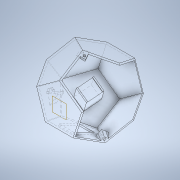
# Autodesk Inventor part: dodecahedron
Saved by Autodesk Inventor 2020.2 (Build 242310000, 310)
## iProperties
Created: 2020-01-17
Part Number: dodecahedron
Material: Generic
Document SubType Name: Modeling
Designer: Bardo91
Density: 1 g/cm^3
Appearance: Default
Author: Bardo91
Autodesk Inventor part; units mm, degrees
ref_plane "YZ Plane" through (0, 0, 0) normal (1, 0, 0) x (0, 1, 0)
ref_plane "XZ Plane" through (0, 0, 0) normal (0, 1, 0) x (-1, 0, 0)
ref_plane "Work Plane1" through (0, 0, 44.5407) normal (0, 0, 1) x (1, 0, 0)
sketch "Sketch2" plane through (0, 0, 44.5407) normal (0, 0, 1) x (1, 0, 0)
  line L0 (0, 34.026) -> (32.3607, 10.5146)
  line L1 (32.3607, 10.5146) -> (20, -27.5276)
  line L2 (20, -27.5276) -> (-20, -27.5276)
  line L3 (-20, -27.5276) -> (-32.3607, 10.5146)
  line L4 (-32.3607, 10.5146) -> (0, 34.026)
  point P0 (0, 0)
  point P1 (0, 0)
  dimension "d2" = 40
  constraints: 10 end point, 1 coincident, 11 other
  measures "d2" distance of L1.end L2.end
loft "Loft1" add profiles "Sketch2" section 2 point at (0, 0, 0)
mirror "Mirror1" about plane through (32.3607, 10.5146, 44.5407) normal (0.809017, -0.2628656, -0.5257311) of "Loft1"
mirror "Mirror2" about plane through (20, -27.5276, 44.5407) normal (0, -0.8506508, -0.5257311) of "Loft1"
mirror "Mirror3" about plane through (-20, -27.5276, 44.5407) normal (-0.809017, -0.2628656, -0.5257311) of "Loft1"
mirror "Mirror4" about plane through (-32.3607, 10.5146, 44.5407) normal (-0.5, 0.688191, -0.5257311) of "Loft1"
mirror "Mirror5" about plane through (0, 34.026, 44.5407) normal (0.5, 0.688191, -0.5257311) of "Loft1"
mirror "Mirror6" about plane through (-52.3607, -17.013, -10.5146) normal (0.309017, -0.4253254, -0.8506508) of "Loft1", "Mirror3"
mirror "Mirror7" about plane through (-52.3607, 17.013, 10.5146) normal (0, 0.5257311, -0.8506508) of "Loft1", "Mirror3"
mirror "Mirror8" about plane through (52.3607, -17.013, -10.5146) normal (0, 0.5257311, -0.8506508) of "Loft1", "Mirror1"
mirror "Mirror9" about plane through (20, 27.5276, -44.5407) normal (-0.809017, -0.2628656, -0.5257311) of "Loft1", "Mirror1", "Mirror8"
shell "Shell1" thickness 2 removed faces 3 at (21.5738, 29.6938, 26.1889) at (39.0273, 17.013, -14.8469) at (39.0273, -5.671, 21.8566)
sketch "Sketch3" plane through (-30.9076, -10.0425, -42.5407) normal (0.5257311, 0.7236068, 0.4472136) x (0.809017, -0.5877853, 0)
  line L0 (19.1019, -26.2916) -> (10.1019, -26.2916)
  line L1 (10.1019, -26.2916) -> (10.1019, -15.2916)
  line L2 (10.1019, -15.2916) -> (28.1019, -15.2916)
  line L3 (28.1019, -15.2916) -> (28.1019, -37.2916)
  line L4 (28.1019, -37.2916) -> (10.1019, -37.2916)
  line L5 (10.1019, -37.2916) -> (10.1019, -26.2916)
  dimension "d8" = 9
  dimension "d9" = 11
  dimension "d10" = 18
  dimension "d11" = 22
  constraints: 12 end point, 4 perpendicular, 1 horizontal, 1 point on line, 1 vertical
  measures "d8" distance of L0.start L0.end
  measures "d9" distance of L0.end L1.end
  measures "d10" distance of L1.end L2.end
  measures "d11" distance of L2.end L3.end
extrude "Extrusion1" add sketch "Sketch3" along normal blind 45
sketch "Sketch4" plane through (-17.9753, -40.0526, -9.1861) normal (0.809017, -0.5877853, 0) x (0.2628656, 0.3618034, -0.8944272)
  line L0 (0, 45) -> (22, 45) projected
  line L1 (11, 45) -> (20.25, 45)
  line L2 (11, 45) -> (1.75, 45)
  line L3 (1.75, 45) -> (1.75, 43)
  line L4 (1.75, 43) -> (20.25, 43)
  line L5 (20.25, 43) -> (20.25, 45)
  point P0 (11, 42.5407)
  dimension "d14" = 9.25
  dimension "d15" = 9.25
  dimension "d16" = 2
  constraints: 10 end point, 3 perpendicular, 2 point on line, 1 midpoint
  measures "d14" distance of L1.start L1.end
  measures "d15" distance of L1.start L2.end
  measures "d16" distance of L2.end L3.end
extrude "Extrusion2" cut sketch "Sketch4" against normal up to surface (18 mm away)
sketch "Sketch5" plane through (-20, -27.5276, 44.5407) normal (0, -0.8944272, 0.4472136) x (1, 0, 0)
  line L0 (20, -27.5276) -> (20, -11.7776)
  line L1 (20, -11.7776) -> (30, -11.7776)
  line L2 (30, -11.7776) -> (30, -43.2776)
  line L3 (30, -43.2776) -> (10, -43.2776)
  line L4 (10, -43.2776) -> (10, -11.7776)
  line L5 (10, -11.7776) -> (20, -11.7776)
  line L6 (30.5, -11.2776) -> (20, -11.2776)
  line L7 (20, -11.2776) -> (9.5, -11.2776)
  line L8 (9.5, -11.2776) -> (9.5, -43.7776)
  line L9 (9.5, -43.7776) -> (30.5, -43.7776)
  line L10 (30.5, -43.7776) -> (30.5, -11.2776)
  dimension "d19" = 15.75
  dimension "d20" = 10
  dimension "d21" = 31.5
  dimension "d22" = 20
  dimension "d25" = 0.5
  constraints: 22 end point, 9 perpendicular, 1 point on line, 1 vertical, 4 other
  measures "d19" distance of L0.start L0.end
  measures "d20" distance of L0.end L1.end
  measures "d21" distance of L1.end L2.end
  measures "d22" distance of L2.end L3.end
  measures "d25" distance between parallel lines of L1 L6
extrude "Extrusion3" cut sketch "Sketch5" against normal up to surface (2 mm away) contours L1 L2 L3 L4 L5 | L10 L9 L8 L7 L6
sketch "Sketch6" plane through (-20, -27.5276, 44.5407) normal (-0.8506508, -0.2763932, 0.4472136) x (0.4253254, 0.1381966, 0.8944272)
  line L0 (0, 0) -> (-38.0423, -12.3607) projected
  line L1 (-27.5276, 20) -> (-19.3486, 22.6575)
  line L2 (-27.1569, 20.1205) -> (-35.336, 17.4629)
  line L3 (-35.336, 17.4629) -> (-35.954, 19.365)
  line L4 (-35.954, 19.365) -> (-19.9666, 24.5597)
  line L5 (-19.9666, 24.5597) -> (-19.3486, 22.6575)
  line L6 (-28.1457, 21.9021) -> (-28.9182, 24.2798)
  line L7 (-28.9182, 24.2798) -> (-24.6385, 25.6703)
  line L8 (-28.9182, 24.2798) -> (-33.198, 22.8892)
  line L9 (-33.198, 22.8892) -> (-32.4254, 20.5115)
  line L10 (-24.6385, 25.6703) -> (-23.8659, 23.2927)
  dimension "d26" = 8.6
  dimension "d27" = 8.6
  dimension "d28" = 2
  dimension "d29" = 2.5
  dimension "d30" = 4.5
  dimension "d31" = 4.5
  constraints: 20 end point, 5 point on line, 4 perpendicular, 3 parallel, 1 collinear
  measures "d26" distance of L1.start L1.end
  measures "d27" distance of L2.start L2.end
  measures "d28" distance of L2.end L3.end
  measures "d29" distance of L6.start L6.end
  measures "d30" distance of L6.end L7.end
  measures "d31" distance of L6.end L8.end
extrude "Extrusion4" cut sketch "Sketch6" against normal up to surface (2 mm away)
sketch "Sketch7" plane through (-30.9076, 10.0425, 42.5407) normal (0.8506508, 0.2763932, -0.4472136) x (-0.5, 0.1624598, -0.8506508)
  line L0 (25.7441, -31.1174) -> (12.1444, -21.2366) projected
  line L1 (12.1444, -21.2366) -> (25.7441, -31.1174)
  line L2 (25.7441, -31.1174) -> (24.5686, -32.7354)
  line L3 (24.5686, -32.7354) -> (10.9688, -22.8547)
  line L4 (10.9688, -22.8547) -> (12.1444, -21.2366)
  point P0 (19.1019, -26.2916)
  dimension "d34" = 2
  constraints: 8 end point, 3 perpendicular, 1 collinear
  measures "d34" distance of L0.start L2.end
extrude "Extrusion5" add sketch "Sketch7" along normal blind 10
chamfer "Chamfer1" distance 10 angle 45 1 edges at (-35.2764, -13.3987, 19.7433)
sketch "Sketch9" plane through (20, -27.5276, 44.5407) normal (0.8506508, -0.2763932, 0.4472136) x (0.4253254, -0.1381966, -0.8944272)
  line L0 (60.1717, 21.9021) -> (37.1882, -9.732) projected
  line L1 (37.1882, -9.732) -> (40.1271, -5.6869)
  line L2 (37.1882, -9.732) -> (32.4329, -8.1869)
  line L3 (37.1882, -9.732) -> (2.2361, 1.6246) projected
  line L4 (32.4329, -8.1869) -> (34.9106, -2.7224)
  line L5 (34.9106, -2.7224) -> (40.1271, -5.6869)
  point P0 (27.5276, 20)
  dimension "d40" = 5
  dimension "d41" = 5
  dimension "d42" = 6
  constraints: 8 end point, 2 point on line
  measures "d40" distance of L0.end L1.end
  measures "d41" distance of L0.end L2.end
  measures "d42" distance of L2.end L4.end
extrude "Extrusion6" add sketch "Sketch9" against normal blind 10
sketch "Sketch10" plane through (32.8097, -41.9226, 11.2786) normal (0.1624598, -0.6708204, -0.7236068) x (-0.8506508, 0.2763932, -0.4472136)
  line L0 (0, 5) -> (10, 5) projected
  line L1 (0, 5) -> (10, 5)
  line L2 (10, 5) -> (10, 0) projected
  line L3 (10, 5) -> (10, 0)
  line L4 (34.4982, -12.5322) -> (0, 0) projected
  line L5 (10, 0) -> (0, 0)
  line L6 (0, 39.1019) -> (0, 5) projected
  line L7 (0, 0) -> (0, 5)
  point P0 (44.5407, 18.3754)
  constraints: 8 end point, 2 perpendicular, 1 collinear, 1 horizontal
extrude "Extrusion7" add sketch "Sketch10" along normal up to surface surface through (22.3649, -30.7827, -19.0248) normal (0.5257311, -0.7236068, -0.4472136)
sketch "Sketch11" plane through (22.7581, -37.0321, 11.0597) normal (-0.4253254, -0.8618034, 0.2763932) x (0.8506508, -0.2763932, 0.4472136)
  line L0 (10, -0.6678) -> (10, 0) projected
  line L1 (0, 0) -> (0, -0.6678) projected
  line L2 (10, 0) -> (0, 0)
  line L3 (0, -5) -> (0, 0) projected
  line L4 (0, 0) -> (0, -5)
  line L5 (10, -5) -> (10, 0) projected
  line L6 (0, -5) -> (10, -5)
  line L7 (10, -5) -> (10, 0)
  point P0 (-34.5407, 13.3754)
  constraints: 8 end point, 2 collinear, 1 horizontal, 1 perpendicular
extrude "Extrusion8" add sketch "Sketch11" along normal up to surface surface through (0, -38.0495, 19.0248) normal (0, -0.8944272, 0.4472136)
sketch "Sketch12" plane through (20, -27.5276, 44.5407) normal (0.8506508, -0.2763932, 0.4472136) x (0.4253254, -0.1381966, -0.8944272)
  line L0 (38.0423, -12.3607) -> (61.5537, 20) projected
  line L1 (34.9106, -2.7224) -> (40.1271, -5.6869) projected
  line L2 (38.0423, -12.3607) -> (34.9106, -2.7224)
  line L3 (38.0423, -12.3607) -> (36.1882, -6.6543)
  circle A0 centre (36.1882, -6.6543) radius 1.5
  point P0 (27.5276, 20)
  dimension "d49" = 6
  dimension "d50" = 3
  constraints: 4 end point, 1 centre point, 1 coincident, 1 point on line
  measures "d49" distance of L0.start L3.end
  measures "d50" diameter of A0
extrude "Extrusion9" cut sketch "Sketch12" against normal up to surface (10 mm away)
sketch "Sketch13" plane through (0, 34.026, 44.5407) normal (0.5257311, 0.7236068, 0.4472136) x (0.809017, -0.5877853, 0)
  line L0 (-9.732, 37.1882) -> (21.9021, 60.1717) projected
  line L1 (-9.732, 37.1882) -> (-5.6869, 40.1271)
  line L2 (-9.732, 37.1882) -> (-8.1869, 32.4329)
  line L3 (1.6246, 2.2361) -> (-9.732, 37.1882) projected
  line L4 (-8.1869, 32.4329) -> (-2.7224, 34.9106)
  line L5 (-5.6869, 40.1271) -> (-2.7224, 34.9106)
  point P0 (20, 27.5276)
  dimension "d53" = 5
  dimension "d54" = 5
  dimension "d55" = 6
  dimension "d56" = 6
  constraints: 8 end point, 2 point on line
  measures "d53" distance of L0.start L1.end
  measures "d54" distance of L0.start L2.end
  measures "d55" distance of L2.end L4.end
  measures "d56" distance of L4.end L1.end
extrude "Extrusion10" add sketch "Sketch13" against normal blind 10
sketch "Sketch14" plane through (5.9472, 51.8868, 8.6499) normal (-0.2628656, 0.6381966, -0.7236068) x (-0.809017, 0.2628656, 0.5257311)
  line L0 (0.6678, 0) -> (0, 0) projected
  line L1 (0, 0) -> (0, -10) projected
  line L2 (0, 0) -> (0, -10)
  line L3 (5, -10) -> (0, -10) projected
  line L4 (0, -10) -> (5, -10)
  line L5 (5, 0) -> (17.5322, -34.4982) projected
  line L6 (5, -10) -> (5, 0)
  line L7 (5, 0) -> (0, 0) projected
  line L8 (5, 0) -> (0, 0)
  point P0 (-13.3754, -44.5407)
  constraints: 8 end point, 3 collinear, 1 perpendicular
extrude "Extrusion11" add sketch "Sketch14" along normal up to surface surface through (0, 38.0495, -19.0248) normal (0, 0.8944272, -0.4472136)
sketch "Sketch15" plane through (-3.3552, 43.3365, 11.0597) normal (-0.8506508, 0.4472136, 0.2763932) x (0, -0.5257311, 0.8506508)
  line L0 (0, 10) -> (-5, 10) projected
  line L1 (-5, 10) -> (0, 10)
  line L2 (0, 10) -> (0, 0) projected
  line L3 (0, 10) -> (0, 0)
  line L4 (0, 0) -> (-5, 0) projected
  line L5 (0, 0) -> (-5, 0)
  line L6 (-5, 0) -> (-5, 10)
  point P0 (13.3754, -34.5407)
  constraints: 8 end point, 3 collinear, 1 perpendicular
extrude "Extrusion12" add sketch "Sketch15" along normal up to surface surface through (-22.3649, 30.7827, 19.0248) normal (-0.5257311, 0.7236068, 0.4472136)
sketch "Sketch16" plane through (0, 34.026, 44.5407) normal (0.5257311, 0.7236068, 0.4472136) x (0.809017, -0.5877853, 0)
  line L0 (0, 0) -> (-12.3607, 38.0423) projected
  line L1 (-5.6869, 40.1271) -> (-2.7224, 34.9106) projected
  line L2 (-12.3607, 38.0423) -> (-2.7224, 34.9106)
  line L3 (20, 61.5537) -> (-12.3607, 38.0423) projected
  line L4 (-12.3607, 38.0423) -> (-6.6543, 36.1882)
  circle A0 centre (-6.6543, 36.1882) radius 1.5
  point P0 (20, 27.5276)
  dimension "d63" = 6
  dimension "d64" = 3
  constraints: 4 end point, 1 centre point, 1 coincident, 1 point on line
  measures "d63" distance of L0.end L4.end
  measures "d64" diameter of A0
extrude "Extrusion13" cut sketch "Sketch16" against normal up to surface (10 mm away)
equation "\"d8\" = 0.5 * d10"
equation "\"d9\" = 0.5 * d11"
body "Solid1"
